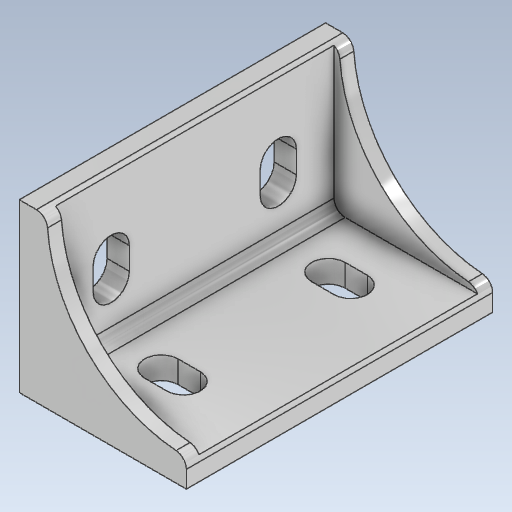
# Autodesk Inventor part: Bracket 3055
Saved by Autodesk Inventor 2020.2 (Build 242310000, 310)
## iProperties
Created: 2019-12-18
Part Number: Bracket 3055
Material: Aluminum 6061, Welded
Document SubType Name: Modeling
Designer: Sunoj
Density: 2.7 g/cm^3
Appearance: Aluminum - Polished
Mass: 33.4325 g
Surface Area: 76.5381 cm^2
Volume: 12.3824 cm^3
Author: Sunoj
Autodesk Inventor part; units mm, degrees
ref_plane "YZ Plane" through (0, 0, 0) normal (1, 0, 0) x (0, 1, 0)
ref_plane "XZ Plane" through (0, 0, 0) normal (0, 1, 0) x (-1, 0, 0)
ref_plane "XY Plane" through (0, 0, 0) normal (0, 0, 1) x (1, 0, 0)
sketch "Sketch1" plane through (0, 0, 0) normal (0, 0, 1) x (1, 0, 0)
  line L0 (0, 0) -> (30, 0)
  line L1 (30, 0) -> (30, 3.0742)
  line L2 (3.0742, 30) -> (0, 30)
  line L3 (0, 30) -> (0, 0)
  line L4 (4, 30) -> (4, 4)
  line L5 (4, 4) -> (30, 4)
  line L6 (4, 30) -> (5, 30)
  line L7 (30, 4) -> (30, 5)
  arc A0 (5.0687, 28.1481) -> (28.1481, 5.0687) centre (30, 30) ccw
  arc A1 (5.0687, 28.1481) -> (3.0742, 30) centre (3.0742, 28) ccw
  arc A2 (30, 3.0742) -> (28.1481, 5.0687) centre (28, 3.0742) ccw
  point P0 (29.7728, 4)
  point P1 (4, 29.7728)
  dimension "d2" = 26
  dimension "d3" = 26
  dimension "d4" = 1
  dimension "d5" = 1
  dimension "d6" = 25
  dimension "d7" = 2
  constraints: 16 end point, 8 point on circle, 4 tangent, 3 centre point, 2 parallel, 2 point on line, 1 equal radius, 1 horizontal, 1 perpendicular
  measures "d2" distance of L5.end L4.end
  measures "d3" distance of L4.end L4.start
  measures "d4" distance of L4.start L6.end
  measures "d5" distance of L5.end L7.end
  measures "d6" radius of A0
  measures "d7" radius of A1
extrude "Extrusion1" add sketch "Sketch1" along normal blind 50 contours L3 L2 A1 L4 L5 A2 L1 L0
extrude "Extrusion2" add sketch "Sketch1" against normal blind 2.5
extrude "Extrusion3" add sketch "Sketch1" along normal blind 2.5 from surface at 50
sketch "Sketch2" plane through (0, 0, -2.5) normal (0, -1, 0) x (1, 0, 0)
  line L0 (30, 0) -> (0, 0) projected
  line L1 (30, 0) -> (15, 0)
  line L2 (15, 0) -> (15, 12.5)
  line L3 (28.1481, 55) -> (5.0687, 55) projected
  line L4 (15, 12.5) -> (15, 42.5)
  line L5 (13, 42.5) -> (17, 42.5) construction
  line L6 (13, 39.5) -> (17, 39.5)
  line L7 (17, 45.5) -> (13, 45.5)
  arc A0 (13, 45.5) -> (13, 39.5) centre (13, 42.5) ccw
  arc A1 (17, 39.5) -> (17, 45.5) centre (17, 42.5) ccw
  line L8 (13, 12.5) -> (17, 12.5) construction
  line L9 (13, 9.5) -> (17, 9.5)
  line L10 (17, 15.5) -> (13, 15.5)
  arc A2 (13, 15.5) -> (13, 9.5) centre (13, 12.5) ccw
  arc A3 (17, 9.5) -> (17, 15.5) centre (17, 12.5) ccw
  point P0 (0, 2.5)
  dimension "d14" = 15
  dimension "d15" = 12.5
  dimension "d16" = 30
  dimension "d17" = 2
  dimension "d18" = 6
  dimension "d19" = 2
  dimension "d20" = 6
  constraints: 22 end point, 8 point on circle, 8 tangent, 4 centre point, 3 midpoint, 3 parallel, 1 horizontal, 1 perpendicular, 1 point on line
  measures "d14" distance of L0.start L1.end
  measures "d15" distance of L1.end L2.end
  measures "d16" distance of L2.end L4.end
  measures "d17" distance of L4.end L5.end
  measures "d18" diameter of A1
  measures "d19" distance of L2.end L8.end
  measures "d20" diameter of A3
extrude "Extrusion4" cut sketch "Sketch2" against normal blind 4
fillet "Fillet1" radius 2 1 edges at (4, 4, 25)
sketch "Sketch3" plane through (0, 0, -2.5) normal (-1, 0, 0) x (0, 0, 1)
  line L0 (0, 0) -> (55, 0) projected
  line L1 (55, 0) -> (55, 15)
  line L2 (55, 5.0687) -> (55, 28.1481) projected
  line L3 (55, 15) -> (42.5, 15)
  line L4 (42.5, 15) -> (12.5, 15)
  line L5 (12.5, 13) -> (12.5, 17) construction
  line L6 (15.75, 13) -> (15.75, 17)
  line L7 (9.25, 17) -> (9.25, 13)
  arc A0 (9.25, 13) -> (15.75, 13) centre (12.5, 13) ccw
  arc A1 (15.75, 17) -> (9.25, 17) centre (12.5, 17) ccw
  line L8 (42.5, 13) -> (42.5, 17) construction
  line L9 (45.75, 13) -> (45.75, 17)
  line L10 (39.25, 17) -> (39.25, 13)
  arc A2 (39.25, 13) -> (45.75, 13) centre (42.5, 13) ccw
  arc A3 (45.75, 17) -> (39.25, 17) centre (42.5, 17) ccw
  dimension "d31" = 15
  dimension "d32" = 12.5
  dimension "d33" = 30
  dimension "d34" = 2
  dimension "d35" = 6.5
  dimension "d36" = 2
  dimension "d37" = 6.5
  constraints: 22 end point, 8 point on circle, 8 tangent, 4 centre point, 2 horizontal, 2 midpoint, 2 parallel, 1 perpendicular, 1 point on line, 1 vertical
  measures "d31" distance of L0.end L1.end
  measures "d32" distance of L1.end L3.end
  measures "d33" distance of L3.end L4.end
  measures "d34" distance of L4.end L5.end
  measures "d35" diameter of A1
  measures "d36" distance of L3.end L8.end
  measures "d37" diameter of A3
extrude "Extrusion5" cut sketch "Sketch3" against normal blind 4
body "Solid1"
